Autodesk Fusion 360 part; units mm, degrees
(part 6 of 7)
  line L307 (64.3585, -53.8636) -> (64.3996, -53.9376)
  line L308 (64.3996, -53.9376) -> (64.4442, -54.0112)
  line L309 (64.4442, -54.0112) -> (64.4922, -54.0844)
  line L310 (64.4922, -54.0844) -> (64.6218, -54.0883)
  line L311 (64.6218, -54.0883) -> (64.7514, -54.0883)
  line L312 (64.7514, -54.0883) -> (64.8809, -54.0844)
  line L313 (64.8809, -54.0844) -> (64.9289, -54.0112)
  line L314 (64.9289, -54.0112) -> (64.9735, -53.9376)
  line L315 (64.9735, -53.9376) -> (65.0146, -53.8636)
  line L316 (65.0146, -53.8636) -> (65.0522, -53.7895)
  line L317 (65.0522, -53.7895) -> (65.0861, -53.7152)
  line L318 (65.0861, -53.7152) -> (65.1162, -53.641)
  line L319 (65.1162, -53.641) -> (65.1424, -53.5668)
  line L320 (65.1424, -53.5668) -> (65.1646, -53.4928)
  line L321 (65.1646, -53.4928) -> (65.1823, -53.4192)
  line L322 (65.1823, -53.4192) -> (65.1951, -53.346)
  line L323 (65.1951, -53.346) -> (65.2023, -53.2736)
  line L324 (65.2023, -53.2736) -> (65.2012, -53.2024)
  line L325 (65.2012, -53.2024) -> (65.1566, -52.9129)
  line L326 (65.1566, -52.9129) -> (65.3224, -52.8827)
  line L327 (65.3224, -52.8827) -> (65.4863, -52.8435)
  line L328 (65.4863, -52.8435) -> (65.6479, -52.7955)
  line L329 (65.6479, -52.7955) -> (65.8065, -52.7387)
  line L330 (65.8065, -52.7387) -> (65.9127, -53.0117)
  line L331 (65.9127, -53.0117) -> (65.9473, -53.074)
  line L332 (65.9473, -53.074) -> (65.9898, -53.1331)
  line L333 (65.9898, -53.1331) -> (66.0375, -53.19)
  line L334 (66.0375, -53.19) -> (66.0896, -53.2449)
  line L335 (66.0896, -53.2449) -> (66.1458, -53.2979)
  line L336 (66.1458, -53.2979) -> (66.2056, -53.3491)
  line L337 (66.2056, -53.3491) -> (66.2688, -53.3983)
  line L338 (66.2688, -53.3983) -> (66.3353, -53.4457)
  line L339 (66.3353, -53.4457) -> (66.4049, -53.4911)
  line L340 (66.4049, -53.4911) -> (66.4775, -53.5346)
  line L341 (66.4775, -53.5346) -> (66.5529, -53.576)
  line L342 (66.5529, -53.576) -> (66.631, -53.6154)
  line L343 (66.631, -53.6154) -> (66.7452, -53.5541)
  line L344 (66.7452, -53.5541) -> (66.8575, -53.4893)
  line L345 (66.8575, -53.4893) -> (66.9677, -53.4211)
  line L346 (66.9677, -53.4211) -> (66.9726, -53.3337)
  line L347 (66.9726, -53.3337) -> (66.9745, -53.2476)
  line L348 (66.9745, -53.2476) -> (66.9731, -53.1631)
  line L349 (66.9731, -53.1631) -> (66.9685, -53.0801)
  line L350 (66.9685, -53.0801) -> (66.9608, -52.9988)
  line L351 (66.9608, -52.9988) -> (66.9497, -52.9194)
  line L352 (66.9497, -52.9194) -> (66.9353, -52.8421)
  line L353 (66.9353, -52.8421) -> (66.9175, -52.7669)
  line L354 (66.9175, -52.7669) -> (66.896, -52.6943)
  line L355 (66.896, -52.6943) -> (66.8706, -52.6245)
  line L356 (66.8706, -52.6245) -> (66.8406, -52.5582)
  line L357 (66.8406, -52.5582) -> (66.804, -52.4971)
  line L358 (66.804, -52.4971) -> (66.6207, -52.2687)
  line L359 (66.6207, -52.2687) -> (66.7492, -52.1597)
  line L360 (66.7492, -52.1597) -> (66.8715, -52.0438)
  line L361 (66.8715, -52.0438) -> (66.9874, -51.9214)
  line L362 (66.9874, -51.9214) -> (67.0964, -51.7929)
  line L363 (67.0964, -51.7929) -> (67.3249, -51.9762)
  line L364 (67.3249, -51.9762) -> (67.386, -52.0128)
  line L365 (67.386, -52.0128) -> (67.4523, -52.0429)
  line L366 (67.4523, -52.0429) -> (67.5221, -52.0683)
  line L367 (67.5221, -52.0683) -> (67.5947, -52.0898)
  line L368 (67.5947, -52.0898) -> (67.6698, -52.1076)
  line L369 (67.6698, -52.1076) -> (67.7472, -52.122)
  line L370 (67.7472, -52.122) -> (67.8266, -52.133)
  line L371 (67.8266, -52.133) -> (67.9079, -52.1408)
  line L372 (67.9079, -52.1408) -> (67.9908, -52.1453)
  line L373 (67.9908, -52.1453) -> (68.0754, -52.1467)
  line L374 (68.0754, -52.1467) -> (68.1614, -52.1449)
  line L375 (68.1614, -52.1449) -> (68.2488, -52.1399)
  line L376 (68.2488, -52.1399) -> (68.317, -52.0297)
  line L377 (68.317, -52.0297) -> (68.3818, -51.9175)
  line L378 (68.3818, -51.9175) -> (68.4432, -51.8033)
  line L379 (68.4432, -51.8033) -> (68.4038, -51.7251)
  line L380 (68.4038, -51.7251) -> (68.3623, -51.6497)
  line L381 (68.3623, -51.6497) -> (68.3189, -51.5771)
  line L382 (68.3189, -51.5771) -> (68.2734, -51.5076)
  line L383 (68.2734, -51.5076) -> (68.2261, -51.4411)
  line L384 (68.2261, -51.4411) -> (68.1768, -51.3778)
  line L385 (68.1768, -51.3778) -> (68.1257, -51.318)
  line L386 (68.1257, -51.318) -> (68.0727, -51.2619)
  line L387 (68.0727, -51.2619) -> (68.0178, -51.2097)
  line L388 (68.0178, -51.2097) -> (67.9609, -51.162)
  line L389 (67.9609, -51.162) -> (67.9017, -51.1196)
  line L390 (67.9017, -51.1196) -> (67.8395, -51.0849)
  line L391 (67.8395, -51.0849) -> (67.5665, -50.9788)
  line L392 (67.5665, -50.9788) -> (67.6233, -50.8201)
  line L393 (67.6233, -50.8201) -> (67.6713, -50.6586)
  line L394 (67.6713, -50.6586) -> (67.7105, -50.4947)
  line L395 (67.7105, -50.4947) -> (67.7406, -50.3289)
  circle A0 centre (64.6866, -49.8588) radius 1.5
extrude "Extrude2''" add sketch "Sketch2 (3)" along normal blind 2 separate body makes body 9 in component "CT idler 3"
combine "Combine1''" operation add target body 8 tool bodies 9 makes body 10 at (67.2226, -49.8588, 43.4) in component "CT idler 3"
ref_plane "WorkPlane1" through (0, 0, 43.4) normal (0, 0, 1) x (1, 0, 0) in component "CT dial wheel (tool body)"
sketch "Sketch1 (5)" plane through (0, 0, 43.4) normal (0, 0, 1) x (1, 0, 0) in component "CT dial wheel (tool body)"
  line L0 (77.5002, -64.378) -> (77.8386, -64.3931)
  line L1 (77.8386, -64.3931) -> (77.9197, -64.3899)
  line L2 (77.9197, -64.3899) -> (78.0011, -64.3809)
  line L3 (78.0011, -64.3809) -> (78.0827, -64.3681)
  line L4 (78.0827, -64.3681) -> (78.1643, -64.3521)
  line L5 (78.1643, -64.3521) -> (78.2461, -64.3334)
  line L6 (78.2461, -64.3334) -> (78.3278, -64.3121)
  line L7 (78.3278, -64.3121) -> (78.4096, -64.2885)
  line L8 (78.4096, -64.2885) -> (78.4914, -64.2626)
  line L9 (78.4914, -64.2626) -> (78.5732, -64.2346)
  line L10 (78.5732, -64.2346) -> (78.6549, -64.2046)
  line L11 (78.6549, -64.2046) -> (78.7366, -64.1726)
  line L12 (78.7366, -64.1726) -> (78.8182, -64.1388)
  line L13 (78.8182, -64.1388) -> (78.8198, -64.0063)
  line L14 (78.8198, -64.0063) -> (78.8198, -63.8737)
  line L15 (78.8198, -63.8737) -> (78.8182, -63.7412)
  line L16 (78.8182, -63.7412) -> (78.7366, -63.7074)
  line L17 (78.7366, -63.7074) -> (78.6549, -63.6754)
  line L18 (78.6549, -63.6754) -> (78.5732, -63.6454)
  line L19 (78.5732, -63.6454) -> (78.4914, -63.6174)
  line L20 (78.4914, -63.6174) -> (78.4096, -63.5915)
  line L21 (78.4096, -63.5915) -> (78.3278, -63.5679)
  line L22 (78.3278, -63.5679) -> (78.2461, -63.5466)
  line L23 (78.2461, -63.5466) -> (78.1643, -63.5279)
  line L24 (78.1643, -63.5279) -> (78.0827, -63.5119)
  line L25 (78.0827, -63.5119) -> (78.0011, -63.4991)
  line L26 (78.0011, -63.4991) -> (77.9197, -63.4901)
  line L27 (77.9197, -63.4901) -> (77.8386, -63.4869)
  line L28 (77.8386, -63.4869) -> (77.5002, -63.502)
  line L29 (77.5002, -63.502) -> (77.4887, -63.2934)
  line L30 (77.4887, -63.2934) -> (77.4727, -63.085)
  line L31 (77.4727, -63.085) -> (77.4522, -62.877)
  line L32 (77.4522, -62.877) -> (77.4274, -62.6695)
  line L33 (77.4274, -62.6695) -> (77.7632, -62.6257)
  line L34 (77.7632, -62.6257) -> (77.8426, -62.6084)
  line L35 (77.8426, -62.6084) -> (77.9212, -62.5854)
  line L36 (77.9212, -62.5854) -> (77.9993, -62.5587)
  line L37 (77.9993, -62.5587) -> (78.0769, -62.5288)
  line L38 (78.0769, -62.5288) -> (78.1542, -62.4961)
  line L39 (78.1542, -62.4961) -> (78.231, -62.461)
  line L40 (78.231, -62.461) -> (78.3074, -62.4235)
  line L41 (78.3074, -62.4235) -> (78.3835, -62.3838)
  line L42 (78.3835, -62.3838) -> (78.4592, -62.342)
  line L43 (78.4592, -62.342) -> (78.5344, -62.2983)
  line L44 (78.5344, -62.2983) -> (78.6093, -62.2526)
  line L45 (78.6093, -62.2526) -> (78.6838, -62.2051)
  line L46 (78.6838, -62.2051) -> (78.6624, -62.0743)
  line L47 (78.6624, -62.0743) -> (78.6394, -61.9438)
  line L48 (78.6394, -61.9438) -> (78.6148, -61.8136)
  line L49 (78.6148, -61.8136) -> (78.5285, -61.7944)
  line L50 (78.5285, -61.7944) -> (78.4425, -61.7771)
  line L51 (78.4425, -61.7771) -> (78.3568, -61.7618)
  line L52 (78.3568, -61.7618) -> (78.2714, -61.7484)
  line L53 (78.2714, -61.7484) -> (78.1864, -61.7371)
  line L54 (78.1864, -61.7371) -> (78.1018, -61.728)
  line L55 (78.1018, -61.728) -> (78.0175, -61.7213)
  line L56 (78.0175, -61.7213) -> (77.9338, -61.717)
  line L57 (77.9338, -61.717) -> (77.8506, -61.7155)
  line L58 (77.8506, -61.7155) -> (77.7681, -61.717)
  line L59 (77.7681, -61.717) -> (77.6863, -61.7223)
  line L60 (77.6863, -61.7223) -> (77.6059, -61.7332)
  line L61 (77.6059, -61.7332) -> (77.2753, -61.8069)
  line L62 (77.2753, -61.8069) -> (77.2277, -61.6034)
  line L63 (77.2277, -61.6034) -> (77.1757, -61.401)
  line L64 (77.1757, -61.401) -> (77.1195, -61.1997)
  line L65 (77.1195, -61.1997) -> (77.059, -60.9997)
  line L66 (77.059, -60.9997) -> (77.3821, -60.8982)
  line L67 (77.3821, -60.8982) -> (77.4573, -60.8674)
  line L68 (77.4573, -60.8674) -> (77.5307, -60.8311)
  line L69 (77.5307, -60.8311) -> (77.603, -60.7912)
  line L70 (77.603, -60.7912) -> (77.6742, -60.7483)
  line L71 (77.6742, -60.7483) -> (77.7446, -60.7027)
  line L72 (77.7446, -60.7027) -> (77.8142, -60.6547)
  line L73 (77.8142, -60.6547) -> (77.8829, -60.6045)
  line L74 (77.8829, -60.6045) -> (77.9509, -60.5523)
  line L75 (77.9509, -60.5523) -> (78.0182, -60.498)
  line L76 (78.0182, -60.498) -> (78.0848, -60.4418)
  line L77 (78.0848, -60.4418) -> (78.1506, -60.3839)
  line L78 (78.1506, -60.3839) -> (78.2157, -60.3241)
  line L79 (78.2157, -60.3241) -> (78.1719, -60.1991)
  line L80 (78.1719, -60.1991) -> (78.1265, -60.0745)
  line L81 (78.1265, -60.0745) -> (78.0797, -59.9506)
  line L82 (78.0797, -59.9506) -> (77.9915, -59.9467)
  line L83 (77.9915, -59.9467) -> (77.9038, -59.9446)
  line L84 (77.9038, -59.9446) -> (77.8167, -59.9443)
  line L85 (77.8167, -59.9443) -> (77.7303, -59.946)
  line L86 (77.7303, -59.946) -> (77.6446, -59.9496)
  line L87 (77.6446, -59.9496) -> (77.5596, -59.9554)
  line L88 (77.5596, -59.9554) -> (77.4755, -59.9634)
  line L89 (77.4755, -59.9634) -> (77.3923, -59.9737)
  line L90 (77.3923, -59.9737) -> (77.3101, -59.9866)
  line L91 (77.3101, -59.9866) -> (77.2291, -60.0025)
  line L92 (77.2291, -60.0025) -> (77.1495, -60.0219)
  line L93 (77.1495, -60.0219) -> (77.0722, -60.0466)
  line L94 (77.0722, -60.0466) -> (76.7594, -60.1766)
  line L95 (76.7594, -60.1766) -> (76.6772, -59.9844)
  line L96 (76.6772, -59.9844) -> (76.5909, -59.7941)
  line L97 (76.5909, -59.7941) -> (76.5006, -59.6057)
  line L98 (76.5006, -59.6057) -> (76.4062, -59.4192)
  line L99 (76.4062, -59.4192) -> (76.7068, -59.2631)
  line L100 (76.7068, -59.2631) -> (76.7755, -59.2198)
  line L101 (76.7755, -59.2198) -> (76.8415, -59.1713)
  line L102 (76.8415, -59.1713) -> (76.9057, -59.1194)
  line L103 (76.9057, -59.1194) -> (76.9685, -59.0648)
  line L104 (76.9685, -59.0648) -> (77.0299, -59.0077)
  line L105 (77.0299, -59.0077) -> (77.09, -58.9483)
  line L106 (77.09, -58.9483) -> (77.149, -58.887)
  line L107 (77.149, -58.887) -> (77.2069, -58.8237)
  line L108 (77.2069, -58.8237) -> (77.2638, -58.7586)
  line L109 (77.2638, -58.7586) -> (77.3195, -58.6917)
  line L110 (77.3195, -58.6917) -> (77.3743, -58.6232)
  line L111 (77.3743, -58.6232) -> (77.428, -58.553)
  line L112 (77.428, -58.553) -> (77.3632, -58.4375)
  line L113 (77.3632, -58.4375) -> (77.2969, -58.3227)
  line L114 (77.2969, -58.3227) -> (77.2293, -58.2088)
  line L115 (77.2293, -58.2088) -> (77.1417, -58.2202)
  line L116 (77.1417, -58.2202) -> (77.0549, -58.2334)
  line L117 (77.0549, -58.2334) -> (76.9691, -58.2483)
  line L118 (76.9691, -58.2483) -> (76.8843, -58.2649)
  line L119 (76.8843, -58.2649) -> (76.8006, -58.2834)
  line L120 (76.8006, -58.2834) -> (76.7179, -58.3038)
  line L121 (76.7179, -58.3038) -> (76.6365, -58.3263)
  line L122 (76.6365, -58.3263) -> (76.5563, -58.3509)
  line L123 (76.5563, -58.3509) -> (76.4776, -58.3779)
  line L124 (76.4776, -58.3779) -> (76.4006, -58.4076)
  line L125 (76.4006, -58.4076) -> (76.3256, -58.4405)
  line L126 (76.3256, -58.4405) -> (76.2537, -58.4783)
  line L127 (76.2537, -58.4783) -> (75.9682, -58.6606)
  line L128 (75.9682, -58.6606) -> (75.8539, -58.4857)
  line L129 (75.8539, -58.4857) -> (75.7359, -58.3132)
  line L130 (75.7359, -58.3132) -> (75.6142, -58.1433)
  line L131 (75.6142, -58.1433) -> (75.4889, -57.9761)
  line L132 (75.4889, -57.9761) -> (75.7578, -57.7702)
  line L133 (75.7578, -57.7702) -> (75.8179, -57.7155)
  line L134 (75.8179, -57.7155) -> (75.8745, -57.6563)
  line L135 (75.8745, -57.6563) -> (75.9288, -57.5941)
  line L136 (75.9288, -57.5941) -> (75.9811, -57.5294)
  line L137 (75.9811, -57.5294) -> (76.0316, -57.4625)
  line L138 (76.0316, -57.4625) -> (76.0806, -57.3936)
  line L139 (76.0806, -57.3936) -> (76.128, -57.3229)
  line L140 (76.128, -57.3229) -> (76.1741, -57.2505)
  line L141 (76.1741, -57.2505) -> (76.2187, -57.1765)
  line L142 (76.2187, -57.1765) -> (76.262, -57.101)
  line L143 (76.262, -57.101) -> (76.3041, -57.024)
  line L144 (76.3041, -57.024) -> (76.3448, -56.9456)
  line L145 (76.3448, -56.9456) -> (76.2609, -56.8431)
  line L146 (76.2609, -56.8431) -> (76.1757, -56.7416)
  line L147 (76.1757, -56.7416) -> (76.0893, -56.6411)
  line L148 (76.0893, -56.6411) -> (76.005, -56.6676)
  line L149 (76.005, -56.6676) -> (75.9219, -56.6956)
  line L150 (75.9219, -56.6956) -> (75.84, -56.7252)
  line L151 (75.84, -56.7252) -> (75.7593, -56.7563)
  line L152 (75.7593, -56.7563) -> (75.6801, -56.7891)
  line L153 (75.6801, -56.7891) -> (75.6022, -56.8235)
  line L154 (75.6022, -56.8235) -> (75.5259, -56.8598)
  line L155 (75.5259, -56.8598) -> (75.4512, -56.8979)
  line L156 (75.4512, -56.8979) -> (75.3784, -56.9382)
  line L157 (75.3784, -56.9382) -> (75.3077, -56.9808)
  line L158 (75.3077, -56.9808) -> (75.2396, -57.0263)
  line L159 (75.2396, -57.0263) -> (75.1753, -57.076)
  line L160 (75.1753, -57.076) -> (74.9259, -57.305)
  line L161 (74.9259, -57.305) -> (74.7829, -57.1526)
  line L162 (74.7829, -57.1526) -> (74.6367, -57.0033)
  line L163 (74.6367, -57.0033) -> (74.4874, -56.8571)
  line L164 (74.4874, -56.8571) -> (74.335, -56.7141)
  line L165 (74.335, -56.7141) -> (74.564, -56.4647)
  line L166 (74.564, -56.4647) -> (74.6137, -56.4004)
  line L167 (74.6137, -56.4004) -> (74.6592, -56.3323)
  line L168 (74.6592, -56.3323) -> (74.7018, -56.2616)
  line L169 (74.7018, -56.2616) -> (74.7421, -56.1888)
  line L170 (74.7421, -56.1888) -> (74.7802, -56.1141)
  line L171 (74.7802, -56.1141) -> (74.8165, -56.0378)
  line L172 (74.8165, -56.0378) -> (74.8509, -55.9599)
  line L173 (74.8509, -55.9599) -> (74.8837, -55.8807)
  line L174 (74.8837, -55.8807) -> (74.9148, -55.8)
  line L175 (74.9148, -55.8) -> (74.9444, -55.7181)
  line L176 (74.9444, -55.7181) -> (74.9724, -55.635)
  line L177 (74.9724, -55.635) -> (74.9989, -55.5507)
  line L178 (74.9989, -55.5507) -> (74.8984, -55.4643)
  line L179 (74.8984, -55.4643) -> (74.7969, -55.3791)
  line L180 (74.7969, -55.3791) -> (74.6944, -55.2952)
  line L181 (74.6944, -55.2952) -> (74.616, -55.3359)
  line L182 (74.616, -55.3359) -> (74.539, -55.378)
  line L183 (74.539, -55.378) -> (74.4635, -55.4213)
  line L184 (74.4635, -55.4213) -> (74.3895, -55.4659)
  line L185 (74.3895, -55.4659) -> (74.3171, -55.512)
  line L186 (74.3171, -55.512) -> (74.2464, -55.5594)
  line L187 (74.2464, -55.5594) -> (74.1775, -55.6084)
  line L188 (74.1775, -55.6084) -> (74.1106, -55.6589)
  line L189 (74.1106, -55.6589) -> (74.0459, -55.7112)
  line L190 (74.0459, -55.7112) -> (73.9837, -55.7655)
  line L191 (73.9837, -55.7655) -> (73.9245, -55.8221)
  line L192 (73.9245, -55.8221) -> (73.8698, -55.8822)
  line L193 (73.8698, -55.8822) -> (73.6639, -56.1511)
  line L194 (73.6639, -56.1511) -> (73.4967, -56.0258)
  line L195 (73.4967, -56.0258) -> (73.3268, -55.9041)
  line L196 (73.3268, -55.9041) -> (73.1543, -55.7861)
  line L197 (73.1543, -55.7861) -> (72.9794, -55.6718)
  line L198 (72.9794, -55.6718) -> (73.1617, -55.3863)
  line L199 (73.1617, -55.3863) -> (73.1995, -55.3144)
  line L200 (73.1995, -55.3144) -> (73.2324, -55.2394)
  line L201 (73.2324, -55.2394) -> (73.2621, -55.1624)
  line L202 (73.2621, -55.1624) -> (73.2891, -55.0837)
  line L203 (73.2891, -55.0837) -> (73.3137, -55.0035)
  line L204 (73.3137, -55.0035) -> (73.3362, -54.9221)
  line L205 (73.3362, -54.9221) -> (73.3566, -54.8394)
  line L206 (73.3566, -54.8394) -> (73.3751, -54.7557)
  line L207 (73.3751, -54.7557) -> (73.3917, -54.6709)
  line L208 (73.3917, -54.6709) -> (73.4066, -54.5851)
  line L209 (73.4066, -54.5851) -> (73.4198, -54.4983)
  line L210 (73.4198, -54.4983) -> (73.4312, -54.4107)
  line L211 (73.4312, -54.4107) -> (73.3173, -54.3431)
  line L212 (73.3173, -54.3431) -> (73.2025, -54.2768)
  line L213 (73.2025, -54.2768) -> (73.087, -54.212)
  line L214 (73.087, -54.212) -> (73.0168, -54.2657)
  line L215 (73.0168, -54.2657) -> (72.9483, -54.3205)
  line L216 (72.9483, -54.3205) -> (72.8814, -54.3762)
  line L217 (72.8814, -54.3762) -> (72.8163, -54.4331)
  line L218 (72.8163, -54.4331) -> (72.753, -54.491)
  line L219 (72.753, -54.491) -> (72.6917, -54.55)
  line L220 (72.6917, -54.55) -> (72.6323, -54.6101)
  line L221 (72.6323, -54.6101) -> (72.5752, -54.6715)
  line L222 (72.5752, -54.6715) -> (72.5206, -54.7343)
  line L223 (72.5206, -54.7343) -> (72.4687, -54.7985)
  line L224 (72.4687, -54.7985) -> (72.4202, -54.8645)
  line L225 (72.4202, -54.8645) -> (72.3769, -54.9332)
  line L226 (72.3769, -54.9332) -> (72.2208, -55.2338)
  line L227 (72.2208, -55.2338) -> (72.0343, -55.1394)
  line L228 (72.0343, -55.1394) -> (71.8459, -55.0491)
  line L229 (71.8459, -55.0491) -> (71.6556, -54.9628)
  line L230 (71.6556, -54.9628) -> (71.4634, -54.8806)
  line L231 (71.4634, -54.8806) -> (71.5934, -54.5678)
  line L232 (71.5934, -54.5678) -> (71.6181, -54.4905)
  line L233 (71.6181, -54.4905) -> (71.6375, -54.4109)
  line L234 (71.6375, -54.4109) -> (71.6534, -54.3299)
  line L235 (71.6534, -54.3299) -> (71.6663, -54.2477)
  line L236 (71.6663, -54.2477) -> (71.6766, -54.1645)
  line L237 (71.6766, -54.1645) -> (71.6846, -54.0804)
  line L238 (71.6846, -54.0804) -> (71.6904, -53.9954)
  line L239 (71.6904, -53.9954) -> (71.694, -53.9097)
  line L240 (71.694, -53.9097) -> (71.6957, -53.8233)
  line L241 (71.6957, -53.8233) -> (71.6954, -53.7362)
  line L242 (71.6954, -53.7362) -> (71.6933, -53.6485)
  line L243 (71.6933, -53.6485) -> (71.6894, -53.5603)
  line L244 (71.6894, -53.5603) -> (71.5655, -53.5135)
  line L245 (71.5655, -53.5135) -> (71.4409, -53.4681)
  line L246 (71.4409, -53.4681) -> (71.3159, -53.4243)
  line L247 (71.3159, -53.4243) -> (71.2561, -53.4894)
  line L248 (71.2561, -53.4894) -> (71.1982, -53.5552)
  line L249 (71.1982, -53.5552) -> (71.142, -53.6218)
  line L250 (71.142, -53.6218) -> (71.0877, -53.6891)
  line L251 (71.0877, -53.6891) -> (71.0355, -53.7571)
  line L252 (71.0355, -53.7571) -> (70.9853, -53.8258)
  line L253 (70.9853, -53.8258) -> (70.9373, -53.8954)
  line L254 (70.9373, -53.8954) -> (70.8917, -53.9658)
  line L255 (70.8917, -53.9658) -> (70.8488, -54.037)
  line L256 (70.8488, -54.037) -> (70.8089, -54.1093)
  line L257 (70.8089, -54.1093) -> (70.7726, -54.1827)
  line L258 (70.7726, -54.1827) -> (70.7418, -54.2579)
  line L259 (70.7418, -54.2579) -> (70.6403, -54.581)
  line L260 (70.6403, -54.581) -> (70.4403, -54.5205)
  line L261 (70.4403, -54.5205) -> (70.239, -54.4643)
  line L262 (70.239, -54.4643) -> (70.0366, -54.4123)
  line L263 (70.0366, -54.4123) -> (69.8331, -54.3647)
  line L264 (69.8331, -54.3647) -> (69.9068, -54.0341)
  line L265 (69.9068, -54.0341) -> (69.9177, -53.9537)
  line L266 (69.9177, -53.9537) -> (69.923, -53.8719)
  line L267 (69.923, -53.8719) -> (69.9245, -53.7894)
  line L268 (69.9245, -53.7894) -> (69.923, -53.7062)
  line L269 (69.923, -53.7062) -> (69.9187, -53.6225)
  line L270 (69.9187, -53.6225) -> (69.912, -53.5382)
  line L271 (69.912, -53.5382) -> (69.9029, -53.4536)
  line L272 (69.9029, -53.4536) -> (69.8916, -53.3686)
  line L273 (69.8916, -53.3686) -> (69.8782, -53.2832)
  line L274 (69.8782, -53.2832) -> (69.8629, -53.1975)
  line L275 (69.8629, -53.1975) -> (69.8456, -53.1115)
  line L276 (69.8456, -53.1115) -> (69.8264, -53.0252)
  line L277 (69.8264, -53.0252) -> (69.6962, -53.0006)
  line L278 (69.6962, -53.0006) -> (69.5657, -52.9776)
  line L279 (69.5657, -52.9776) -> (69.4349, -52.9562)
  line L280 (69.4349, -52.9562) -> (69.3874, -53.0307)
  line L281 (69.3874, -53.0307) -> (69.3417, -53.1056)
  line L282 (69.3417, -53.1056) -> (69.298, -53.1808)
  line L283 (69.298, -53.1808) -> (69.2562, -53.2565)
  line L284 (69.2562, -53.2565) -> (69.2165, -53.3326)
  line L285 (69.2165, -53.3326) -> (69.179, -53.409)
  line L286 (69.179, -53.409) -> (69.1439, -53.4858)
  line L287 (69.1439, -53.4858) -> (69.1112, -53.5631)
  line L288 (69.1112, -53.5631) -> (69.0813, -53.6407)
  line L289 (69.0813, -53.6407) -> (69.0546, -53.7188)
  line L290 (69.0546, -53.7188) -> (69.0316, -53.7974)
  line L291 (69.0316, -53.7974) -> (69.0143, -53.8768)
  line L292 (69.0143, -53.8768) -> (68.9705, -54.2126)
  line L293 (68.9705, -54.2126) -> (68.763, -54.1878)
  line L294 (68.763, -54.1878) -> (68.555, -54.1673)
  line L295 (68.555, -54.1673) -> (68.3466, -54.1513)
  line L296 (68.3466, -54.1513) -> (68.138, -54.1398)
  line L297 (68.138, -54.1398) -> (68.1531, -53.8014)
  line L298 (68.1531, -53.8014) -> (68.1499, -53.7203)
  line L299 (68.1499, -53.7203) -> (68.1409, -53.6389)
  line L300 (68.1409, -53.6389) -> (68.1281, -53.5573)
  line L301 (68.1281, -53.5573) -> (68.1121, -53.4757)
  line L302 (68.1121, -53.4757) -> (68.0934, -53.3939)
  line L303 (68.0934, -53.3939) -> (68.0721, -53.3122)
  line L304 (68.0721, -53.3122) -> (68.0485, -53.2304)
  line L305 (68.0485, -53.2304) -> (68.0226, -53.1486)
  line L306 (68.0226, -53.1486) -> (67.9946, -53.0668)
  line L307 (67.9946, -53.0668) -> (67.9646, -52.9851)
  line L308 (67.9646, -52.9851) -> (67.9326, -52.9034)
  line L309 (67.9326, -52.9034) -> (67.8988, -52.8218)
  line L310 (67.8988, -52.8218) -> (67.7663, -52.8202)
  line L311 (67.7663, -52.8202) -> (67.6337, -52.8202)
  line L312 (67.6337, -52.8202) -> (67.5012, -52.8218)
  line L313 (67.5012, -52.8218) -> (67.4674, -52.9034)
  line L314 (67.4674, -52.9034) -> (67.4354, -52.9851)
  line L315 (67.4354, -52.9851) -> (67.4054, -53.0668)
  line L316 (67.4054, -53.0668) -> (67.3774, -53.1486)
  line L317 (67.3774, -53.1486) -> (67.3515, -53.2304)
  line L318 (67.3515, -53.2304) -> (67.3279, -53.3122)
  line L319 (67.3279, -53.3122) -> (67.3066, -53.3939)
  line L320 (67.3066, -53.3939) -> (67.2879, -53.4757)
  line L321 (67.2879, -53.4757) -> (67.2719, -53.5573)
  line L322 (67.2719, -53.5573) -> (67.2591, -53.6389)
  line L323 (67.2591, -53.6389) -> (67.2501, -53.7203)
  line L324 (67.2501, -53.7203) -> (67.2469, -53.8014)
  line L325 (67.2469, -53.8014) -> (67.262, -54.1398)
  line L326 (67.262, -54.1398) -> (67.0534, -54.1513)
  line L327 (67.0534, -54.1513) -> (66.845, -54.1673)
  line L328 (66.845, -54.1673) -> (66.637, -54.1878)
  line L329 (66.637, -54.1878) -> (66.4295, -54.2126)
  line L330 (66.4295, -54.2126) -> (66.3857, -53.8768)
  line L331 (66.3857, -53.8768) -> (66.3684, -53.7974)
  line L332 (66.3684, -53.7974) -> (66.3454, -53.7188)
  line L333 (66.3454, -53.7188) -> (66.3187, -53.6407)
  line L334 (66.3187, -53.6407) -> (66.2888, -53.5631)
  line L335 (66.2888, -53.5631) -> (66.2561, -53.4858)
  line L336 (66.2561, -53.4858) -> (66.221, -53.409)
  line L337 (66.221, -53.409) -> (66.1835, -53.3326)
  line L338 (66.1835, -53.3326) -> (66.1438, -53.2565)
  line L339 (66.1438, -53.2565) -> (66.102, -53.1808)
  line L340 (66.102, -53.1808) -> (66.0583, -53.1056)
  line L341 (66.0583, -53.1056) -> (66.0126, -53.0307)
  line L342 (66.0126, -53.0307) -> (65.9651, -52.9562)
  line L343 (65.9651, -52.9562) -> (65.8343, -52.9776)
  line L344 (65.8343, -52.9776) -> (65.7038, -53.0006)
  line L345 (65.7038, -53.0006) -> (65.5736, -53.0252)
  line L346 (65.5736, -53.0252) -> (65.5544, -53.1115)
  line L347 (65.5544, -53.1115) -> (65.5371, -53.1975)
  line L348 (65.5371, -53.1975) -> (65.5218, -53.2832)
  line L349 (65.5218, -53.2832) -> (65.5084, -53.3686)
  line L350 (65.5084, -53.3686) -> (65.4971, -53.4536)
  line L351 (65.4971, -53.4536) -> (65.488, -53.5382)
  line L352 (65.488, -53.5382) -> (65.4813, -53.6225)
  line L353 (65.4813, -53.6225) -> (65.477, -53.7062)
  line L354 (65.477, -53.7062) -> (65.4755, -53.7894)
  line L355 (65.4755, -53.7894) -> (65.477, -53.8719)
  line L356 (65.477, -53.8719) -> (65.4823, -53.9537)
  line L357 (65.4823, -53.9537) -> (65.4932, -54.0341)
  line L358 (65.4932, -54.0341) -> (65.5669, -54.3647)
  line L359 (65.5669, -54.3647) -> (65.3634, -54.4123)
  line L360 (65.3634, -54.4123) -> (65.161, -54.4643)
  line L361 (65.161, -54.4643) -> (64.9597, -54.5205)
  line L362 (64.9597, -54.5205) -> (64.7597, -54.581)
  line L363 (64.7597, -54.581) -> (64.6582, -54.2579)
  line L364 (64.6582, -54.2579) -> (64.6274, -54.1827)
  line L365 (64.6274, -54.1827) -> (64.5911, -54.1093)
  line L366 (64.5911, -54.1093) -> (64.5512, -54.037)
  line L367 (64.5512, -54.037) -> (64.5083, -53.9658)
  line L368 (64.5083, -53.9658) -> (64.4627, -53.8954)
  line L369 (64.4627, -53.8954) -> (64.4147, -53.8258)
  line L370 (64.4147, -53.8258) -> (64.3645, -53.7571)
  line L371 (64.3645, -53.7571) -> (64.3123, -53.6891)
  line L372 (64.3123, -53.6891) -> (64.258, -53.6218)
  line L373 (64.258, -53.6218) -> (64.2018, -53.5552)
  line L374 (64.2018, -53.5552) -> (64.1439, -53.4894)
  line L375 (64.1439, -53.4894) -> (64.0841, -53.4243)
  line L376 (64.0841, -53.4243) -> (63.9591, -53.4681)
  line L377 (63.9591, -53.4681) -> (63.8345, -53.5135)
  line L378 (63.8345, -53.5135) -> (63.7106, -53.5603)
  line L379 (63.7106, -53.5603) -> (63.7067, -53.6485)
  line L380 (63.7067, -53.6485) -> (63.7046, -53.7362)
  line L381 (63.7046, -53.7362) -> (63.7043, -53.8233)
  line L382 (63.7043, -53.8233) -> (63.706, -53.9097)
  line L383 (63.706, -53.9097) -> (63.7096, -53.9954)
  line L384 (63.7096, -53.9954) -> (63.7154, -54.0804)
  line L385 (63.7154, -54.0804) -> (63.7234, -54.1645)
  line L386 (63.7234, -54.1645) -> (63.7337, -54.2477)
  line L387 (63.7337, -54.2477) -> (63.7466, -54.3299)
  line L388 (63.7466, -54.3299) -> (63.7625, -54.4109)
  line L389 (63.7625, -54.4109) -> (63.7819, -54.4905)
  line L390 (63.7819, -54.4905) -> (63.8066, -54.5678)
  line L391 (63.8066, -54.5678) -> (63.9366, -54.8806)
  line L392 (63.9366, -54.8806) -> (63.7444, -54.9628)
  line L393 (63.7444, -54.9628) -> (63.5541, -55.0491)
  line L394 (63.5541, -55.0491) -> (63.3657, -55.1394)
  line L395 (63.3657, -55.1394) -> (63.1792, -55.2338)
  line L396 (63.1792, -55.2338) -> (63.0231, -54.9332)
  line L397 (63.0231, -54.9332) -> (62.9798, -54.8645)
  line L398 (62.9798, -54.8645) -> (62.9313, -54.7985)
  line L399 (62.9313, -54.7985) -> (62.8794, -54.7343)
  line L400 (62.8794, -54.7343) -> (62.8248, -54.6715)
  line L401 (62.8248, -54.6715) -> (62.7677, -54.6101)
  line L402 (62.7677, -54.6101) -> (62.7083, -54.55)
  line L403 (62.7083, -54.55) -> (62.647, -54.491)
  line L404 (62.647, -54.491) -> (62.5837, -54.4331)
  line L405 (62.5837, -54.4331) -> (62.5186, -54.3762)
  line L406 (62.5186, -54.3762) -> (62.4517, -54.3205)
  line L407 (62.4517, -54.3205) -> (62.3832, -54.2657)
  line L408 (62.3832, -54.2657) -> (62.313, -54.212)
  line L409 (62.313, -54.212) -> (62.1975, -54.2768)
  line L410 (62.1975, -54.2768) -> (62.0827, -54.3431)
  line L411 (62.0827, -54.3431) -> (61.9688, -54.4107)
  line L412 (61.9688, -54.4107) -> (61.9802, -54.4983)
  line L413 (61.9802, -54.4983) -> (61.9934, -54.5851)
  line L414 (61.9934, -54.5851) -> (62.0083, -54.6709)
  line L415 (62.0083, -54.6709) -> (62.0249, -54.7557)
  line L416 (62.0249, -54.7557) -> (62.0434, -54.8394)
  line L417 (62.0434, -54.8394) -> (62.0638, -54.9221)
  line L418 (62.0638, -54.9221) -> (62.0863, -55.0035)
  line L419 (62.0863, -55.0035) -> (62.1109, -55.0837)
  line L420 (62.1109, -55.0837) -> (62.1379, -55.1624)
  line L421 (62.1379, -55.1624) -> (62.1676, -55.2394)
  line L422 (62.1676, -55.2394) -> (62.2005, -55.3144)
  line L423 (62.2005, -55.3144) -> (62.2383, -55.3863)
  line L424 (62.2383, -55.3863) -> (62.4206, -55.6718)
  line L425 (62.4206, -55.6718) -> (62.2457, -55.7861)
  line L426 (62.2457, -55.7861) -> (62.0732, -55.9041)
  line L427 (62.0732, -55.9041) -> (61.9033, -56.0258)
  line L428 (61.9033, -56.0258) -> (61.7361, -56.1511)
  line L429 (61.7361, -56.1511) -> (61.5302, -55.8822)
  line L430 (61.5302, -55.8822) -> (61.4755, -55.8221)
  line L431 (61.4755, -55.8221) -> (61.4163, -55.7655)
  line L432 (61.4163, -55.7655) -> (61.3541, -55.7112)
  line L433 (61.3541, -55.7112) -> (61.2894, -55.6589)
  line L434 (61.2894, -55.6589) -> (61.2225, -55.6084)
  line L435 (61.2225, -55.6084) -> (61.1536, -55.5594)
  line L436 (61.1536, -55.5594) -> (61.0829, -55.512)
  line L437 (61.0829, -55.512) -> (61.0105, -55.4659)
  line L438 (61.0105, -55.4659) -> (60.9365, -55.4213)
  line L439 (60.9365, -55.4213) -> (60.861, -55.378)
  line L440 (60.861, -55.378) -> (60.784, -55.3359)
  line L441 (60.784, -55.3359) -> (60.7056, -55.2952)
  line L442 (60.7056, -55.2952) -> (60.6031, -55.3791)
  line L443 (60.6031, -55.3791) -> (60.5016, -55.4643)
  line L444 (60.5016, -55.4643) -> (60.4011, -55.5507)
  line L445 (60.4011, -55.5507) -> (60.4276, -55.635)
  line L446 (60.4276, -55.635) -> (60.4556, -55.7181)
  line L447 (60.4556, -55.7181) -> (60.4852, -55.8)
  line L448 (60.4852, -55.8) -> (60.5163, -55.8807)
  line L449 (60.5163, -55.8807) -> (60.5491, -55.9599)
  line L450 (60.5491, -55.9599) -> (60.5835, -56.0378)
  line L451 (60.5835, -56.0378) -> (60.6198, -56.1141)
  line L452 (60.6198, -56.1141) -> (60.6579, -56.1888)
  line L453 (60.6579, -56.1888) -> (60.6982, -56.2616)
  line L454 (60.6982, -56.2616) -> (60.7408, -56.3323)
  line L455 (60.7408, -56.3323) -> (60.7863, -56.4004)
  line L456 (60.7863, -56.4004) -> (60.836, -56.4647)
  line L457 (60.836, -56.4647) -> (61.065, -56.7141)
  line L458 (61.065, -56.7141) -> (60.9126, -56.8571)
  line L459 (60.9126, -56.8571) -> (60.7633, -57.0033)
  line L460 (60.7633, -57.0033) -> (60.6171, -57.1526)
  line L461 (60.6171, -57.1526) -> (60.4741, -57.305)
  line L462 (60.4741, -57.305) -> (60.2247, -57.076)
  line L463 (60.2247, -57.076) -> (60.1604, -57.0263)
  line L464 (60.1604, -57.0263) -> (60.0923, -56.9808)
  line L465 (60.0923, -56.9808) -> (60.0216, -56.9382)
  line L466 (60.0216, -56.9382) -> (59.9488, -56.8979)
  line L467 (59.9488, -56.8979) -> (59.8741, -56.8598)
  line L468 (59.8741, -56.8598) -> (59.7978, -56.8235)
  line L469 (59.7978, -56.8235) -> (59.7199, -56.7891)
  line L470 (59.7199, -56.7891) -> (59.6407, -56.7563)
  line L471 (59.6407, -56.7563) -> (59.56, -56.7252)
  line L472 (59.56, -56.7252) -> (59.4781, -56.6956)
  line L473 (59.4781, -56.6956) -> (59.395, -56.6676)
  line L474 (59.395, -56.6676) -> (59.3107, -56.6411)
  line L475 (59.3107, -56.6411) -> (59.2243, -56.7416)
  line L476 (59.2243, -56.7416) -> (59.1391, -56.8431)
  line L477 (59.1391, -56.8431) -> (59.0552, -56.9456)
  line L478 (59.0552, -56.9456) -> (59.0959, -57.024)
  line L479 (59.0959, -57.024) -> (59.138, -57.101)
  line L480 (59.138, -57.101) -> (59.1813, -57.1765)
  line L481 (59.1813, -57.1765) -> (59.2259, -57.2505)
  line L482 (59.2259, -57.2505) -> (59.272, -57.3229)
  line L483 (59.272, -57.3229) -> (59.3194, -57.3936)
  line L484 (59.3194, -57.3936) -> (59.3684, -57.4625)
  line L485 (59.3684, -57.4625) -> (59.4189, -57.5294)
  line L486 (59.4189, -57.5294) -> (59.4712, -57.5941)
  line L487 (59.4712, -57.5941) -> (59.5255, -57.6563)
  line L488 (59.5255, -57.6563) -> (59.5821, -57.7155)
  line L489 (59.5821, -57.7155) -> (59.6422, -57.7702)
  line L490 (59.6422, -57.7702) -> (59.9111, -57.9761)
  line L491 (59.9111, -57.9761) -> (59.7858, -58.1433)
  line L492 (59.7858, -58.1433) -> (59.6641, -58.3132)
  line L493 (59.6641, -58.3132) -> (59.5461, -58.4857)
  line L494 (59.5461, -58.4857) -> (59.4318, -58.6606)
  line L495 (59.4318, -58.6606) -> (59.1463, -58.4783)
  line L496 (59.1463, -58.4783) -> (59.0744, -58.4405)
  line L497 (59.0744, -58.4405) -> (58.9994, -58.4076)
  line L498 (58.9994, -58.4076) -> (58.9224, -58.3779)
  line L499 (58.9224, -58.3779) -> (58.8437, -58.3509)
  line L500 (58.8437, -58.3509) -> (58.7635, -58.3263)
  line L501 (58.7635, -58.3263) -> (58.6821, -58.3038)
  line L502 (58.6821, -58.3038) -> (58.5994, -58.2834)
  line L503 (58.5994, -58.2834) -> (58.5157, -58.2649)
  line L504 (58.5157, -58.2649) -> (58.4309, -58.2483)
  line L505 (58.4309, -58.2483) -> (58.3451, -58.2334)
  line L506 (58.3451, -58.2334) -> (58.2583, -58.2202)
  line L507 (58.2583, -58.2202) -> (58.1707, -58.2088)
  line L508 (58.1707, -58.2088) -> (58.1031, -58.3227)
  line L509 (58.1031, -58.3227) -> (58.0368, -58.4375)
  line L510 (58.0368, -58.4375) -> (57.972, -58.553)
  line L511 (57.972, -58.553) -> (58.0257, -58.6232)
  line L512 (58.0257, -58.6232) -> (58.0805, -58.6917)
  line L513 (58.0805, -58.6917) -> (58.1362, -58.7586)
  line L514 (58.1362, -58.7586) -> (58.1931, -58.8237)
  line L515 (58.1931, -58.8237) -> (58.251, -58.887)
  line L516 (58.251, -58.887) -> (58.31, -58.9483)
  line L517 (58.31, -58.9483) -> (58.3701, -59.0077)
  line L518 (58.3701, -59.0077) -> (58.4315, -59.0648)
  line L519 (58.4315, -59.0648) -> (58.4943, -59.1194)
  line L520 (58.4943, -59.1194) -> (58.5585, -59.1713)
  line L521 (58.5585, -59.1713) -> (58.6245, -59.2198)
  line L522 (58.6245, -59.2198) -> (58.6932, -59.2631)
  line L523 (58.6932, -59.2631) -> (58.9938, -59.4192)
  line L524 (58.9938, -59.4192) -> (58.8994, -59.6057)
  line L525 (58.8994, -59.6057) -> (58.8091, -59.7941)
  line L526 (58.8091, -59.7941) -> (58.7228, -59.9844)
  line L527 (58.7228, -59.9844) -> (58.6406, -60.1766)
  line L528 (58.6406, -60.1766) -> (58.3278, -60.0466)
  line L529 (58.3278, -60.0466) -> (58.2505, -60.0219)
  line L530 (58.2505, -60.0219) -> (58.1709, -60.0025)
  line L531 (58.1709, -60.0025) -> (58.0899, -59.9866)
  line L532 (58.0899, -59.9866) -> (58.0077, -59.9737)
  line L533 (58.0077, -59.9737) -> (57.9245, -59.9634)
  line L534 (57.9245, -59.9634) -> (57.8404, -59.9554)
  line L535 (57.8404, -59.9554) -> (57.7554, -59.9496)
  line L536 (57.7554, -59.9496) -> (57.6697, -59.946)
  line L537 (57.6697, -59.946) -> (57.5833, -59.9443)
  line L538 (57.5833, -59.9443) -> (57.4962, -59.9446)
  line L539 (57.4962, -59.9446) -> (57.4085, -59.9467)
  line L540 (57.4085, -59.9467) -> (57.3203, -59.9506)
  line L541 (57.3203, -59.9506) -> (57.2735, -60.0745)
  line L542 (57.2735, -60.0745) -> (57.2281, -60.1991)
  line L543 (57.2281, -60.1991) -> (57.1843, -60.3241)
  line L544 (57.1843, -60.3241) -> (57.2494, -60.3839)
  line L545 (57.2494, -60.3839) -> (57.3152, -60.4418)
  line L546 (57.3152, -60.4418) -> (57.3818, -60.498)
  line L547 (57.3818, -60.498) -> (57.4491, -60.5523)
  line L548 (57.4491, -60.5523) -> (57.5171, -60.6045)
  line L549 (57.5171, -60.6045) -> (57.5858, -60.6547)
  line L550 (57.5858, -60.6547) -> (57.6554, -60.7027)
  line L551 (57.6554, -60.7027) -> (57.7258, -60.7483)
  line L552 (57.7258, -60.7483) -> (57.797, -60.7912)
  line L553 (57.797, -60.7912) -> (57.8693, -60.8311)
  line L554 (57.8693, -60.8311) -> (57.9427, -60.8674)
  line L555 (57.9427, -60.8674) -> (58.0179, -60.8982)
  line L556 (58.0179, -60.8982) -> (58.341, -60.9997)
  line L557 (58.341, -60.9997) -> (58.2805, -61.1997)
  line L558 (58.2805, -61.1997) -> (58.2243, -61.401)
  line L559 (58.2243, -61.401) -> (58.1723, -61.6034)
  line L560 (58.1723, -61.6034) -> (58.1247, -61.8069)
  line L561 (58.1247, -61.8069) -> (57.7941, -61.7332)
  line L562 (57.7941, -61.7332) -> (57.7137, -61.7223)
  line L563 (57.7137, -61.7223) -> (57.6319, -61.717)
  line L564 (57.6319, -61.717) -> (57.5494, -61.7155)
  line L565 (57.5494, -61.7155) -> (57.4662, -61.717)
  line L566 (57.4662, -61.717) -> (57.3825, -61.7213)
  line L567 (57.3825, -61.7213) -> (57.2982, -61.728)
  line L568 (57.2982, -61.728) -> (57.2136, -61.7371)
  line L569 (57.2136, -61.7371) -> (57.1286, -61.7484)
  line L570 (57.1286, -61.7484) -> (57.0432, -61.7618)
  line L571 (57.0432, -61.7618) -> (56.9575, -61.7771)
  line L572 (56.9575, -61.7771) -> (56.8715, -61.7944)
  line L573 (56.8715, -61.7944) -> (56.7852, -61.8136)
  line L574 (56.7852, -61.8136) -> (56.7606, -61.9438)
  line L575 (56.7606, -61.9438) -> (56.7376, -62.0743)
  line L576 (56.7376, -62.0743) -> (56.7162, -62.2051)
  line L577 (56.7162, -62.2051) -> (56.7907, -62.2526)
  line L578 (56.7907, -62.2526) -> (56.8656, -62.2983)
  line L579 (56.8656, -62.2983) -> (56.9408, -62.342)
  line L580 (56.9408, -62.342) -> (57.0165, -62.3838)
  line L581 (57.0165, -62.3838) -> (57.0926, -62.4235)
  line L582 (57.0926, -62.4235) -> (57.169, -62.461)
  line L583 (57.169, -62.461) -> (57.2458, -62.4961)
  line L584 (57.2458, -62.4961) -> (57.3231, -62.5288)
  line L585 (57.3231, -62.5288) -> (57.4007, -62.5587)
  line L586 (57.4007, -62.5587) -> (57.4788, -62.5854)
  line L587 (57.4788, -62.5854) -> (57.5574, -62.6084)
  line L588 (57.5574, -62.6084) -> (57.6368, -62.6257)
  line L589 (57.6368, -62.6257) -> (57.9726, -62.6695)
  line L590 (57.9726, -62.6695) -> (57.9478, -62.877)
  line L591 (57.9478, -62.877) -> (57.9273, -63.085)
  line L592 (57.9273, -63.085) -> (57.9113, -63.2934)
  line L593 (57.9113, -63.2934) -> (57.8998, -63.502)
  line L594 (57.8998, -63.502) -> (57.5614, -63.4869)
  line L595 (57.5614, -63.4869) -> (57.4803, -63.4901)
  line L596 (57.4803, -63.4901) -> (57.3989, -63.4991)
  line L597 (57.3989, -63.4991) -> (57.3173, -63.5119)
  line L598 (57.3173, -63.5119) -> (57.2357, -63.5279)
  line L599 (57.2357, -63.5279) -> (57.1539, -63.5466)
  line L600 (57.1539, -63.5466) -> (57.0722, -63.5679)
  line L601 (57.0722, -63.5679) -> (56.9904, -63.5915)
  line L602 (56.9904, -63.5915) -> (56.9086, -63.6174)
  line L603 (56.9086, -63.6174) -> (56.8268, -63.6454)
  line L604 (56.8268, -63.6454) -> (56.7451, -63.6754)
  line L605 (56.7451, -63.6754) -> (56.6634, -63.7074)
  line L606 (56.6634, -63.7074) -> (56.5818, -63.7412)
  line L607 (56.5818, -63.7412) -> (56.5802, -63.8737)
  line L608 (56.5802, -63.8737) -> (56.5802, -64.0063)
  line L609 (56.5802, -64.0063) -> (56.5818, -64.1388)
  line L610 (56.5818, -64.1388) -> (56.6634, -64.1726)
  line L611 (56.6634, -64.1726) -> (56.7451, -64.2046)
  line L612 (56.7451, -64.2046) -> (56.8268, -64.2346)
  line L613 (56.8268, -64.2346) -> (56.9086, -64.2626)
  line L614 (56.9086, -64.2626) -> (56.9904, -64.2885)
  line L615 (56.9904, -64.2885) -> (57.0722, -64.3121)
  line L616 (57.0722, -64.3121) -> (57.1539, -64.3334)
  line L617 (57.1539, -64.3334) -> (57.2357, -64.3521)
  line L618 (57.2357, -64.3521) -> (57.3173, -64.3681)
  line L619 (57.3173, -64.3681) -> (57.3989, -64.3809)
  line L620 (57.3989, -64.3809) -> (57.4803, -64.3899)
  line L621 (57.4803, -64.3899) -> (57.5614, -64.3931)
  line L622 (57.5614, -64.3931) -> (57.8998, -64.378)
  line L623 (57.8998, -64.378) -> (57.9113, -64.5866)
  line L624 (57.9113, -64.5866) -> (57.9273, -64.795)
  line L625 (57.9273, -64.795) -> (57.9478, -65.003)
  line L626 (57.9478, -65.003) -> (57.9726, -65.2105)
  line L627 (57.9726, -65.2105) -> (57.6368, -65.2543)
  line L628 (57.6368, -65.2543) -> (57.5574, -65.2716)
  line L629 (57.5574, -65.2716) -> (57.4788, -65.2946)
  line L630 (57.4788, -65.2946) -> (57.4007, -65.3213)
  line L631 (57.4007, -65.3213) -> (57.3231, -65.3512)
  line L632 (57.3231, -65.3512) -> (57.2458, -65.3839)
  line L633 (57.2458, -65.3839) -> (57.169, -65.419)
  line L634 (57.169, -65.419) -> (57.0926, -65.4565)
  line L635 (57.0926, -65.4565) -> (57.0165, -65.4962)
  line L636 (57.0165, -65.4962) -> (56.9408, -65.538)
  line L637 (56.9408, -65.538) -> (56.8656, -65.5817)
  line L638 (56.8656, -65.5817) -> (56.7907, -65.6274)
  line L639 (56.7907, -65.6274) -> (56.7162, -65.6749)
  line L640 (56.7162, -65.6749) -> (56.7376, -65.8057)
  line L641 (56.7376, -65.8057) -> (56.7606, -65.9362)
  line L642 (56.7606, -65.9362) -> (56.7852, -66.0664)
  line L643 (56.7852, -66.0664) -> (56.8715, -66.0856)
  line L644 (56.8715, -66.0856) -> (56.9575, -66.1029)
  line L645 (56.9575, -66.1029) -> (57.0432, -66.1182)
  line L646 (57.0432, -66.1182) -> (57.1286, -66.1316)
  line L647 (57.1286, -66.1316) -> (57.2136, -66.1429)
  line L648 (57.2136, -66.1429) -> (57.2982, -66.152)
  line L649 (57.2982, -66.152) -> (57.3825, -66.1587)
  line L650 (57.3825, -66.1587) -> (57.4662, -66.163)
  line L651 (57.4662, -66.163) -> (57.5494, -66.1645)
  line L652 (57.5494, -66.1645) -> (57.6319, -66.163)
  line L653 (57.6319, -66.163) -> (57.7137, -66.1577)
  line L654 (57.7137, -66.1577) -> (57.7941, -66.1468)
  line L655 (57.7941, -66.1468) -> (58.1247, -66.0731)
  line L656 (58.1247, -66.0731) -> (58.1723, -66.2766)
  line L657 (58.1723, -66.2766) -> (58.2243, -66.479)
  line L658 (58.2243, -66.479) -> (58.2805, -66.6803)
  line L659 (58.2805, -66.6803) -> (58.341, -66.8803)
  line L660 (58.341, -66.8803) -> (58.0179, -66.9818)
  line L661 (58.0179, -66.9818) -> (57.9427, -67.0126)
  line L662 (57.9427, -67.0126) -> (57.8693, -67.0489)
  line L663 (57.8693, -67.0489) -> (57.797, -67.0888)
  line L664 (57.797, -67.0888) -> (57.7258, -67.1317)
  line L665 (57.7258, -67.1317) -> (57.6554, -67.1773)
  line L666 (57.6554, -67.1773) -> (57.5858, -67.2253)
  line L667 (57.5858, -67.2253) -> (57.5171, -67.2755)
  line L668 (57.5171, -67.2755) -> (57.4491, -67.3277)
  line L669 (57.4491, -67.3277) -> (57.3818, -67.382)
  line L670 (57.3818, -67.382) -> (57.3152, -67.4382)
  line L671 (57.3152, -67.4382) -> (57.2494, -67.4961)
  line L672 (57.2494, -67.4961) -> (57.1843, -67.5559)
  line L673 (57.1843, -67.5559) -> (57.2281, -67.6809)
  line L674 (57.2281, -67.6809) -> (57.2735, -67.8055)
  line L675 (57.2735, -67.8055) -> (57.3203, -67.9294)
  line L676 (57.3203, -67.9294) -> (57.4085, -67.9333)
  line L677 (57.4085, -67.9333) -> (57.4962, -67.9354)
  line L678 (57.4962, -67.9354) -> (57.5833, -67.9357)
  line L679 (57.5833, -67.9357) -> (57.6697, -67.934)
  line L680 (57.6697, -67.934) -> (57.7554, -67.9304)
  line L681 (57.7554, -67.9304) -> (57.8404, -67.9246)
  line L682 (57.8404, -67.9246) -> (57.9245, -67.9166)
  line L683 (57.9245, -67.9166) -> (58.0077, -67.9063)
  line L684 (58.0077, -67.9063) -> (58.0899, -67.8934)
  line L685 (58.0899, -67.8934) -> (58.1709, -67.8775)
  line L686 (58.1709, -67.8775) -> (58.2505, -67.8581)
  line L687 (58.2505, -67.8581) -> (58.3278, -67.8334)
  line L688 (58.3278, -67.8334) -> (58.6406, -67.7034)
  line L689 (58.6406, -67.7034) -> (58.7228, -67.8956)
  line L690 (58.7228, -67.8956) -> (58.8091, -68.0859)
  line L691 (58.8091, -68.0859) -> (58.8994, -68.2743)
  line L692 (58.8994, -68.2743) -> (58.9938, -68.4608)
  line L693 (58.9938, -68.4608) -> (58.6932, -68.6169)
  line L694 (58.6932, -68.6169) -> (58.6245, -68.6602)
  line L695 (58.6245, -68.6602) -> (58.5585, -68.7087)
  line L696 (58.5585, -68.7087) -> (58.4943, -68.7606)
  line L697 (58.4943, -68.7606) -> (58.4315, -68.8152)
  line L698 (58.4315, -68.8152) -> (58.3701, -68.8723)
  line L699 (58.3701, -68.8723) -> (58.31, -68.9317)
  line L700 (58.31, -68.9317) -> (58.251, -68.993)
  line L701 (58.251, -68.993) -> (58.1931, -69.0563)
  line L702 (58.1931, -69.0563) -> (58.1362, -69.1214)
  line L703 (58.1362, -69.1214) -> (58.0805, -69.1883)
  line L704 (58.0805, -69.1883) -> (58.0257, -69.2568)
  line L705 (58.0257, -69.2568) -> (57.972, -69.327)
  line L706 (57.972, -69.327) -> (58.0368, -69.4425)
  line L707 (58.0368, -69.4425) -> (58.1031, -69.5573)
  line L708 (58.1031, -69.5573) -> (58.1707, -69.6712)
  line L709 (58.1707, -69.6712) -> (58.2583, -69.6598)
  line L710 (58.2583, -69.6598) -> (58.3451, -69.6466)
  line L711 (58.3451, -69.6466) -> (58.4309, -69.6317)
  line L712 (58.4309, -69.6317) -> (58.5157, -69.6151)
  line L713 (58.5157, -69.6151) -> (58.5994, -69.5966)
  line L714 (58.5994, -69.5966) -> (58.6821, -69.5762)
  line L715 (58.6821, -69.5762) -> (58.7635, -69.5537)
  line L716 (58.7635, -69.5537) -> (58.8437, -69.5291)
  line L717 (58.8437, -69.5291) -> (58.9224, -69.5021)
  line L718 (58.9224, -69.5021) -> (58.9994, -69.4724)
  line L719 (58.9994, -69.4724) -> (59.0744, -69.4395)
  line L720 (59.0744, -69.4395) -> (59.1463, -69.4017)
  line L721 (59.1463, -69.4017) -> (59.4318, -69.2194)
  line L722 (59.4318, -69.2194) -> (59.5461, -69.3943)
  line L723 (59.5461, -69.3943) -> (59.6641, -69.5668)
  line L724 (59.6641, -69.5668) -> (59.7858, -69.7367)
  line L725 (59.7858, -69.7367) -> (59.9111, -69.9039)
  line L726 (59.9111, -69.9039) -> (59.6422, -70.1098)
  line L727 (59.6422, -70.1098) -> (59.5821, -70.1645)
  line L728 (59.5821, -70.1645) -> (59.5255, -70.2237)
  line L729 (59.5255, -70.2237) -> (59.4712, -70.2859)
  line L730 (59.4712, -70.2859) -> (59.4189, -70.3506)
  line L731 (59.4189, -70.3506) -> (59.3684, -70.4175)
  line L732 (59.3684, -70.4175) -> (59.3194, -70.4864)
  line L733 (59.3194, -70.4864) -> (59.272, -70.5571)
  line L734 (59.272, -70.5571) -> (59.2259, -70.6295)
  line L735 (59.2259, -70.6295) -> (59.1813, -70.7035)
  line L736 (59.1813, -70.7035) -> (59.138, -70.779)
  line L737 (59.138, -70.779) -> (59.0959, -70.856)
  line L738 (59.0959, -70.856) -> (59.0552, -70.9344)
  line L739 (59.0552, -70.9344) -> (59.1391, -71.0369)
  line L740 (59.1391, -71.0369) -> (59.2243, -71.1384)
  line L741 (59.2243, -71.1384) -> (59.3107, -71.2389)
  line L742 (59.3107, -71.2389) -> (59.395, -71.2124)
  line L743 (59.395, -71.2124) -> (59.4781, -71.1844)
  line L744 (59.4781, -71.1844) -> (59.56, -71.1548)
  line L745 (59.56, -71.1548) -> (59.6407, -71.1237)
  line L746 (59.6407, -71.1237) -> (59.7199, -71.0909)
  line L747 (59.7199, -71.0909) -> (59.7978, -71.0565)
  line L748 (59.7978, -71.0565) -> (59.8741, -71.0202)
  line L749 (59.8741, -71.0202) -> (59.9488, -70.9821)
  line L750 (59.9488, -70.9821) -> (60.0216, -70.9418)
  line L751 (60.0216, -70.9418) -> (60.0923, -70.8992)
  line L752 (60.0923, -70.8992) -> (60.1604, -70.8537)
  line L753 (60.1604, -70.8537) -> (60.2247, -70.804)
  line L754 (60.2247, -70.804) -> (60.4741, -70.575)
  line L755 (60.4741, -70.575) -> (60.6171, -70.7274)
  line L756 (60.6171, -70.7274) -> (60.7633, -70.8767)
  line L757 (60.7633, -70.8767) -> (60.9126, -71.0229)
  line L758 (60.9126, -71.0229) -> (61.065, -71.1659)
  line L759 (61.065, -71.1659) -> (60.836, -71.4153)
  line L760 (60.836, -71.4153) -> (60.7863, -71.4796)
  line L761 (60.7863, -71.4796) -> (60.7408, -71.5477)
  line L762 (60.7408, -71.5477) -> (60.6982, -71.6184)
  line L763 (60.6982, -71.6184) -> (60.6579, -71.6912)
  line L764 (60.6579, -71.6912) -> (60.6198, -71.7659)
  line L765 (60.6198, -71.7659) -> (60.5835, -71.8422)
  line L766 (60.5835, -71.8422) -> (60.5491, -71.9201)
  line L767 (60.5491, -71.9201) -> (60.5163, -71.9993)
  line L768 (60.5163, -71.9993) -> (60.4852, -72.08)
  line L769 (60.4852, -72.08) -> (60.4556, -72.1619)
  line L770 (60.4556, -72.1619) -> (60.4276, -72.245)
  line L771 (60.4276, -72.245) -> (60.4011, -72.3293)
  line L772 (60.4011, -72.3293) -> (60.5016, -72.4157)
  line L773 (60.5016, -72.4157) -> (60.6031, -72.5009)
  line L774 (60.6031, -72.5009) -> (60.7056, -72.5848)
  line L775 (60.7056, -72.5848) -> (60.784, -72.5441)
  line L776 (60.784, -72.5441) -> (60.861, -72.502)
  line L777 (60.861, -72.502) -> (60.9365, -72.4587)
  line L778 (60.9365, -72.4587) -> (61.0105, -72.4141)
  line L779 (61.0105, -72.4141) -> (61.0829, -72.368)
  line L780 (61.0829, -72.368) -> (61.1536, -72.3206)
  line L781 (61.1536, -72.3206) -> (61.2225, -72.2716)
  line L782 (61.2225, -72.2716) -> (61.2894, -72.2211)
  line L783 (61.2894, -72.2211) -> (61.3541, -72.1688)
  line L784 (61.3541, -72.1688) -> (61.4163, -72.1145)
  line L785 (61.4163, -72.1145) -> (61.4755, -72.0579)
  line L786 (61.4755, -72.0579) -> (61.5302, -71.9978)
  line L787 (61.5302, -71.9978) -> (61.7361, -71.7289)
  line L788 (61.7361, -71.7289) -> (61.9033, -71.8542)
  line L789 (61.9033, -71.8542) -> (62.0732, -71.9759)
  line L790 (62.0732, -71.9759) -> (62.2457, -72.0939)
  line L791 (62.2457, -72.0939) -> (62.4206, -72.2082)
  line L792 (62.4206, -72.2082) -> (62.2383, -72.4937)
  line L793 (62.2383, -72.4937) -> (62.2005, -72.5656)
  line L794 (62.2005, -72.5656) -> (62.1676, -72.6406)
  line L795 (62.1676, -72.6406) -> (62.1379, -72.7176)
  line L796 (62.1379, -72.7176) -> (62.1109, -72.7963)
  line L797 (62.1109, -72.7963) -> (62.0863, -72.8765)
  line L798 (62.0863, -72.8765) -> (62.0638, -72.9579)
  line L799 (62.0638, -72.9579) -> (62.0434, -73.0406)
  line L800 (62.0434, -73.0406) -> (62.0249, -73.1243)
  line L801 (62.0249, -73.1243) -> (62.0083, -73.2091)
  line L802 (62.0083, -73.2091) -> (61.9934, -73.2949)
  line L803 (61.9934, -73.2949) -> (61.9802, -73.3817)
  line L804 (61.9802, -73.3817) -> (61.9688, -73.4693)
  line L805 (61.9688, -73.4693) -> (62.0827, -73.5369)
  line L806 (62.0827, -73.5369) -> (62.1975, -73.6032)
  line L807 (62.1975, -73.6032) -> (62.313, -73.668)
  line L808 (62.313, -73.668) -> (62.3832, -73.6143)
  line L809 (62.3832, -73.6143) -> (62.4517, -73.5595)
  line L810 (62.4517, -73.5595) -> (62.5186, -73.5038)
  line L811 (62.5186, -73.5038) -> (62.5837, -73.4469)
  line L812 (62.5837, -73.4469) -> (62.647, -73.389)
  line L813 (62.647, -73.389) -> (62.7083, -73.33)
  line L814 (62.7083, -73.33) -> (62.7677, -73.2699)
  line L815 (62.7677, -73.2699) -> (62.8248, -73.2085)
  line L816 (62.8248, -73.2085) -> (62.8794, -73.1457)